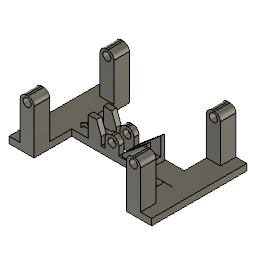
foot (Autodesk Fusion 360 design; units mm, degrees)
part number: 2025-10-24-15-34-12-718
Autodesk Fusion 360 part; units mm, degrees
sketch "Sketch1" plane through (0, 0, 0) normal (0, 0, 1) x (1, 0, 0)
  line L0 (0, 0) -> (180.34, 0)
  line L1 (180.34, 0) -> (180.34, 120.65)
  line L2 (180.34, 120.65) -> (0, 120.65)
  line L3 (0, 120.65) -> (0, 0)
  line L4 (43.18, 0) -> (43.18, 47.625)
  line L5 (43.18, 47.625) -> (137.16, 47.625)
  line L6 (137.16, 47.625) -> (137.16, 0)
  line L7 (43.18, 120.65) -> (43.18, 73.025)
  line L8 (43.18, 73.025) -> (137.16, 73.025)
  line L9 (137.16, 73.025) -> (137.16, 120.65)
  dimension "d1" = 180.34
  dimension "d2" = 120.65
  dimension "d3" = 43.18
  dimension "d4" = 43.18
  dimension "d5" = 43.18
  dimension "d6" = 43.18
  dimension "d8" = 47.625
  dimension "d9" = 47.625
  dimension "d10" = 25.4
  constraint horizontal L0
  constraint vertical L1
  constraint horizontal L2
  constraint vertical L3
  constraint coincident L0.start L3.end
  constraint coincident L0 L4.start
  constraint perpendicular L0 L4
  constraint perpendicular L4 L5
  constraint coincident L0 L6.end
  constraint perpendicular L0 L6
  constraint coincident L2 L7.start
  constraint perpendicular L2 L7
  constraint perpendicular L7 L8
  constraint coincident L2 L9.end
  constraint perpendicular L2 L9
  measures "d1" distance of L0.start L0.end
  measures "d2" distance of L0.start L2.end
  measures "d3" distance of L0.start L4.start
  measures "d4" distance of L0.end L6.end
  measures "d5" distance of L2.end L7.start
  measures "d6" distance of L1.end L9.end
  measures "d8" distance of L8.end L9.end
  measures "d9" distance of L5.end L6.end
  measures "d10" distance of L5.end L8.end
extrude "Extrude1" add sketch "Sketch1" along normal blind 3.175 contours L0 L1 L2 L3 L4 L5 L6 L7 L8 L9
sketch "Sketch2" plane through (0, 0, 3.175) normal (0, 0, 1) x (-1, 0, 0)
  line L0 (-43.18, -120.65) -> (0, -120.65)
  line L1 (0, -120.65) -> (0, 0)
  line L2 (0, 0) -> (-43.18, 0)
  line L3 (-43.18, 0) -> (-43.18, -47.625)
  line L4 (-43.18, -47.625) -> (-137.16, -47.625)
  line L5 (-137.16, -47.625) -> (-137.16, 0)
  line L6 (-137.16, 0) -> (-180.34, 0)
  line L7 (-180.34, 0) -> (-180.34, -120.65)
  line L8 (-180.34, -120.65) -> (-137.16, -120.65)
  line L9 (-137.16, -120.65) -> (-137.16, -73.025)
  line L10 (-137.16, -73.025) -> (-43.18, -73.025)
  line L11 (-43.18, -73.025) -> (-43.18, -120.65)
  line L12 (-73.66, -73.025) -> (-73.66, -47.625)
  line L13 (-91.44, -47.625) -> (-91.44, -73.025)
  dimension "d13" = 30.48
  dimension "d14" = 45.72
  constraint coincident L10 L12.start
  constraint coincident L4 L12.end
  constraint perpendicular L4 L12
  constraint coincident L4 L13.start
  constraint coincident L10 L13.end
  constraint perpendicular L10 L13
  measures "d13" distance of L3.end L12.end
  measures "d14" distance of L4.end L13.start
extrude "Extrude2" add sketch "Sketch2" along normal blind 41.275 contours L4 L10 L12 L13
sketch "Sketch3" plane through (0, 0, 3.175) normal (0, 0, 1) x (-1, 0, 0)
  line L0 (-73.66, -47.625) -> (-73.66, -73.025)
  line L1 (-73.66, -73.025) -> (-43.18, -73.025)
  line L2 (-43.18, -73.025) -> (-43.18, -120.65)
  line L3 (-43.18, -120.65) -> (0, -120.65)
  line L4 (0, -120.65) -> (0, 0)
  line L5 (0, 0) -> (-43.18, 0)
  line L6 (-43.18, 0) -> (-43.18, -47.625)
  line L7 (-43.18, -47.625) -> (-73.66, -47.625)
  line L8 (-31.75, -120.65) -> (-13.97, -120.65)
  line L9 (-13.97, -120.65) -> (-13.97, -100.965)
  line L10 (-13.97, -100.965) -> (-31.75, -100.965)
  line L11 (-31.75, -100.965) -> (-31.75, -120.65)
  line L12 (-31.75, 0) -> (-13.97, 0)
  line L13 (-13.97, 0) -> (-13.97, -19.685)
  line L14 (-13.97, -19.685) -> (-31.75, -19.685)
  line L15 (-31.75, -19.685) -> (-31.75, 0)
  dimension "d18" = 19.685
  dimension "d20" = 19.685
  dimension "d108" = 17.78
  dimension "d109" = 11.43
  dimension "d110" = 17.78
  dimension "d111" = 11.43
  dimension "d113" = 19.685
  constraint horizontal L8
  constraint vertical L9
  constraint horizontal L10
  constraint vertical L11
  constraint horizontal L12
  constraint vertical L13
  constraint horizontal L14
  constraint vertical L15
  constraint coincident L3 L8.start
  measures "d18" distance of L8.start L10.end
  measures "d20" distance of L12.start L14.end
  measures "d108" distance of L9 L11
  measures "d109" distance of L2.end L11
  measures "d110" distance of L13 L15
  measures "d111" distance of L6 L15
  measures "d113" distance of L5 L14
sketch "Sketch4" plane through (0, 0, 3.175) normal (0, 0, 1) x (-1, 0, 0)
  line L0 (-91.44, -73.025) -> (-91.44, -47.625)
  line L1 (-91.44, -47.625) -> (-137.16, -47.625)
  line L2 (-137.16, -47.625) -> (-137.16, 0)
  line L3 (-137.16, 0) -> (-180.34, 0)
  line L4 (-180.34, 0) -> (-180.34, -120.65)
  line L5 (-180.34, -120.65) -> (-137.16, -120.65)
  line L6 (-137.16, -120.65) -> (-137.16, -73.025)
  line L7 (-137.16, -73.025) -> (-91.44, -73.025)
  line L8 (-148.59, -120.65) -> (-166.37, -120.65)
  line L9 (-166.37, -120.65) -> (-166.37, -100.965)
  line L10 (-166.37, -100.965) -> (-148.59, -100.965)
  line L11 (-148.59, 0) -> (-166.37, 0)
  line L12 (-166.37, 0) -> (-166.37, -19.685)
  line L13 (-166.37, -19.685) -> (-148.59, -19.685)
  line L14 (-148.59, -19.685) -> (-148.59, 0)
  line L15 (-148.59, -100.965) -> (-148.59, -120.65)
  dimension "d21" = 17.78
  dimension "d22" = 19.685
  dimension "d95" = 11.43
  dimension "d96" = 17.78
  dimension "d98" = 19.685
  dimension "d99" = 11.43
  constraint horizontal L8
  constraint vertical L9
  constraint horizontal L10
  constraint horizontal L11
  constraint vertical L12
  constraint horizontal L13
  constraint coincident L5 L8.start
  constraint perpendicular L8 L15
  constraint coincident L3 L11.start
  constraint perpendicular L3 L14
  measures "d21" distance of L8.start L8.end
  measures "d22" distance of L8.start L10.end
  measures "d95" distance of L6 L10.end
  measures "d96" distance of L11.start L11.end
  measures "d98" distance of L11.start L13.end
  measures "d99" distance of L2.end L11.start
extrude "Extrude3" add sketch "Sketch3" sketch "Sketch4" along normal blind 41.275 contours L5 L12 L13 L14 L15 | L3 L8 L9 L10 L11 of sketch 2 contours L5 L8 L9 L10 L15 | L3 L11 L12 L13 L14
sketch "Sketch5" plane through (0, 0, 3.175) normal (0, 0, 1) x (-1, 0, 0)
  line L0 (-166.37, -19.685) -> (-166.37, 0)
  line L1 (-166.37, 0) -> (-180.34, 0)
  line L2 (-180.34, 0) -> (-180.34, -120.65)
  line L3 (-180.34, -120.65) -> (-166.37, -120.65)
  line L4 (-166.37, -120.65) -> (-166.37, -100.965)
  line L5 (-166.37, -100.965) -> (-148.59, -100.965)
  line L6 (-137.16, -120.65) -> (-137.16, -73.025)
  line L7 (-137.16, -73.025) -> (-91.44, -73.025)
  line L8 (-91.44, -73.025) -> (-91.44, -47.625)
  line L9 (-91.44, -47.625) -> (-137.16, -47.625)
  line L10 (-137.16, -47.625) -> (-137.16, 0)
  line L11 (-148.59, -19.685) -> (-166.37, -19.685)
  line L12 (-137.16, 0) -> (-158.6586, 0)
  line L13 (-158.6586, 0) -> (-158.6586, -47.6125)
  line L14 (-158.6586, -47.6125) -> (-137.16, -47.6125)
  line L15 (-137.16, -47.6125) -> (-137.16, 0)
  line L16 (-166.37, -100.965) -> (-137.16, -100.965)
  line L17 (-137.16, -100.965) -> (-137.16, -73.025)
  line L18 (-137.16, -73.025) -> (-166.37, -73.025)
  line L19 (-166.37, -73.025) -> (-166.37, -100.965)
  line L20 (-148.59, -100.965) -> (-148.59, -120.65)
  line L21 (-148.59, -120.65) -> (-137.16, -120.65)
  line L22 (-137.16, 0) -> (-148.59, 0)
  line L23 (-148.59, 0) -> (-148.59, -19.685)
  constraint horizontal L12
  constraint vertical L13
  constraint horizontal L14
  constraint vertical L15
  constraint coincident L10.end L12.start
  constraint horizontal L16
  constraint vertical L17
  constraint horizontal L18
  constraint vertical L19
  constraint coincident L6.end L7.start
  constraint coincident L4.end L5.start
sketch "Sketch6" plane through (0, 0, 3.175) normal (0, 0, 1) x (-1, 0, 0)
  line L0 (-13.97, -100.965) -> (-13.97, -120.65)
  line L1 (-13.97, -120.65) -> (0, -120.65)
  line L2 (0, -120.65) -> (0, 0)
  line L3 (0, 0) -> (-13.97, 0)
  line L4 (-13.97, 0) -> (-13.97, -19.685)
  line L5 (-13.97, -19.685) -> (-31.75, -19.685)
  line L6 (-31.75, -19.685) -> (-31.75, 0)
  line L7 (-43.18, -47.625) -> (-73.66, -47.625)
  line L8 (-73.66, -47.625) -> (-73.66, -73.025)
  line L9 (-73.66, -73.025) -> (-43.18, -73.025)
  line L10 (-43.18, -73.025) -> (-43.18, -120.65)
  line L11 (-31.75, -100.965) -> (-13.97, -100.965)
  line L12 (-13.97, -19.685) -> (-31.75, -19.685)
  line L13 (-31.75, -19.685) -> (-31.75, 0)
  line L14 (-31.75, 0) -> (-13.97, 0)
  line L15 (-13.97, 0) -> (-13.97, -19.685)
  line L16 (-13.97, -100.965) -> (-43.18, -100.965)
  line L17 (-43.18, -100.965) -> (-43.18, -73.025)
  line L18 (-43.18, -73.025) -> (-13.97, -73.025)
  line L19 (-13.97, -73.025) -> (-13.97, -100.965)
  line L20 (-31.75, 0) -> (-43.18, 0)
  line L21 (-43.18, 0) -> (-43.18, -47.625)
  line L22 (-43.18, -120.65) -> (-31.75, -120.65)
  line L23 (-31.75, -120.65) -> (-31.75, -100.965)
  constraint horizontal L12
  constraint vertical L13
  constraint horizontal L14
  constraint vertical L15
  constraint coincident L6.end L13.end
  constraint coincident L4.end L5.start
  constraint horizontal L16
  constraint vertical L17
  constraint horizontal L18
  constraint vertical L19
  constraint coincident L9.end L10.start
  constraint coincident L0.start L11.end
extrude "Extrude4" cut sketch "Sketch6" sketch "Sketch5" against normal blind 5.08 contours L10 L11 L16 L17 L18 L19 | L4 L5 L6 L12 L13 L14 L15 of sketch 2 contours L11 L12 L13 L23 | L10 L11 L12 L13 L14 L15 L22 L23 | L5 L6 L16 L17 L18 L19
hole "Hole1" at (82.55, 73.025, 13.335) direction (0, -1, 0) diameter 10.16 depth 30.48 tip angle 118
extrude "Extrude5" add 4 faces at (154.5167, 114.0883, 44.45) (160.4433, 13.1233, 44.45) (25.8233, 6.5617, 44.45) (19.8967, 107.5267, 44.45) along direction (0, 0, 1) blind 14.605
hole "Hole2" at (157.48, 120.65, 51.435) direction (0, -1, 0) diameter 10.16 depth 135.89 tip angle 118
hole "Hole3" at (22.86, 120.65, 51.435) direction (0, -1, 0) diameter 10.16 depth 135.89 tip angle 118
extrude "Extrude6" cut 1 faces at (79.5867, 64.5583, 44.45) along direction (0, 0, -1) blind 22.86
sketch "Sketch7" plane through (0, 0, 21.59) normal (0, 0, 1) x (-1, 0, 0)
  line L0 (-91.44, -47.625) -> (-91.44, -73.025)
  line L1 (-91.44, -73.025) -> (-73.66, -73.025)
  line L2 (-73.66, -73.025) -> (-73.66, -47.625)
  line L3 (-73.66, -47.625) -> (-91.44, -47.625)
  line L4 (-91.44, -53.975) -> (-73.66, -53.975)
  line L5 (-73.66, -53.975) -> (-73.66, -66.675)
  line L6 (-73.66, -66.675) -> (-91.44, -66.675)
  line L7 (-91.44, -66.675) -> (-91.44, -53.975)
  dimension "d48" = 6.35
  dimension "d49" = 6.35
  constraint horizontal L4
  constraint vertical L5
  constraint horizontal L6
  constraint vertical L7
  constraint coincident L2 L5.end
  constraint coincident L0 L4.start
  measures "d48" distance of L3 L4
  measures "d49" distance of L1 L6
extrude "Extrude7" cut sketch "Sketch7" against normal blind 22.86 contours L0 L2 L4 L5 L6 L7
fillet "Fillet1" radius 3.175 1 edges at (73.66, 60.325, 3.175)
fillet "Fillet2" radius 3.175 1 edges at (91.44, 60.325, 3.175)
fillet "Fillet3" radius 7.62 11 edges at (166.37, 9.8425, 59.055) (31.75, 9.8425, 59.055) (31.75, 110.8075, 59.055) (166.37, 110.8075, 59.055) (91.44, 69.85, 21.59) (91.44, 50.8, 21.59) (73.66, 50.8, 21.59) (73.66, 69.85, 21.59) (13.97, 110.8075, 59.055) (13.97, 9.8425, 59.055) (148.59, 9.8425, 59.055)
sketch "Sketch8" plane through (0, 0, 3.175) normal (0, 0, 1) x (-1, 0, 0)
  line L0 (-70.485, -66.675) -> (-73.66, -66.675)
  line L1 (-73.66, -66.675) -> (-73.66, -73.025)
  line L2 (-73.66, -73.025) -> (-13.97, -73.025)
  line L3 (-13.97, -73.025) -> (-13.97, -100.965)
  line L4 (-13.97, -100.965) -> (-13.97, -120.65)
  line L5 (-13.97, -120.65) -> (0, -120.65)
  line L6 (0, -120.65) -> (0, 0)
  line L7 (0, 0) -> (-13.97, 0)
  line L8 (-43.18, -47.625) -> (-73.66, -47.625)
  line L9 (-73.66, -47.625) -> (-73.66, -53.975)
  line L10 (-73.66, -53.975) -> (-70.485, -53.975)
  line L11 (-70.485, -53.975) -> (-70.485, -66.675)
  line L12 (-45.085, -58.3924) -> (-45.085, -62.2024)
  line L13 (-45.085, -62.2024) -> (-36.195, -62.2024)
  line L14 (-36.195, -62.2024) -> (-36.195, -65.7584)
  line L15 (-36.195, -65.7584) -> (-30.732, -60.1732)
  line L16 (-30.732, -60.1732) -> (-36.195, -54.8297)
  line L17 (-36.195, -54.8297) -> (-36.195, -58.3924)
  line L18 (-36.195, -58.3924) -> (-45.085, -58.3924)
  line L19 (-13.97, 0) -> (-13.97, -19.685)
  line L20 (-13.97, -19.685) -> (-31.75, -19.685)
  line L21 (-31.75, -19.685) -> (-31.75, 0)
  line L22 (-31.75, 0) -> (-43.18, 0)
  line L23 (-43.18, 0) -> (-43.18, -47.625)
  dimension "d58" = 4.4726
  dimension "d59" = 3.81
  dimension "d60" = 3.5627
  dimension "d61" = 3.556
  dimension "d62" = 4.4174
  dimension "d75" = 25.4
  constraint parallel L9 L12
  constraint perpendicular L12 L13
  constraint perpendicular L13 L14
  constraint perpendicular L15 L16
  constraint parallel L14 L17
  constraint perpendicular L12 L18
  measures "d58" vertical distance of L0.start L12.end
  measures "d59" distance of L13 L18
  measures "d60" distance of L16.end L17.end
  measures "d61" distance of L13.end L14.end
  measures "d62" vertical distance of L10.end L12.start
  measures "d75" distance of L11 L12.start
extrude "Extrude8" cut sketch "Sketch8" against normal blind 0.508 contours L12 L13 L14 L15 L16 L17 L18
sketch "Sketch9" plane through (0, 0, 3.175) normal (0, 0, 1) x (-1, 0, 0)
  line L0 (-94.615, -53.975) -> (-91.44, -53.975)
  line L1 (-91.44, -53.975) -> (-91.44, -47.625)
  line L2 (-91.44, -47.625) -> (-137.16, -47.625)
  line L3 (-137.16, -47.625) -> (-137.16, -47.6125)
  line L4 (-137.16, -47.6125) -> (-158.6586, -47.6125)
  line L5 (-158.6586, -47.6125) -> (-158.6586, -19.685)
  line L6 (-166.37, -19.685) -> (-166.37, 0)
  line L7 (-166.37, 0) -> (-180.34, 0)
  line L8 (-180.34, 0) -> (-180.34, -120.65)
  line L9 (-180.34, -120.65) -> (-166.37, -120.65)
  line L10 (-166.37, -120.65) -> (-166.37, -100.965)
  line L11 (-166.37, -100.965) -> (-166.37, -73.025)
  line L12 (-166.37, -73.025) -> (-91.44, -73.025)
  line L13 (-91.44, -73.025) -> (-91.44, -66.675)
  line L14 (-91.44, -66.675) -> (-94.615, -66.675)
  line L15 (-94.615, -66.675) -> (-94.615, -53.975)
  line L16 (-107.315, -66.675) -> (-94.615, -66.675)
  line L17 (-94.615, -66.675) -> (-94.615, -53.975)
  line L18 (-94.615, -53.975) -> (-107.315, -53.975)
  line L19 (-107.315, -53.975) -> (-107.315, -66.675)
  line L20 (-158.6586, -19.685) -> (-166.37, -19.685)
  dimension "d65" = 12.7
  dimension "d66" = 12.7
  constraint horizontal L16
  constraint vertical L17
  constraint horizontal L18
  constraint vertical L19
  constraint coincident L0.start L15.end
  measures "d65" distance of L17 L19
  measures "d66" distance of L14.end L0.start
extrude "Extrude9" add sketch "Sketch9" along normal blind 3.7084 contours L15 L16 L17 L18 L19
extrude "Extrude10" cut 1 faces at (103.0817, 58.2083, 6.8834) along direction (0, 0, -1) blind 0.0508
sketch "Sketch10" plane through (0, 66.675, 0) normal (0, 1, 0) x (-1, 0, 0)
  line L0 (-94.615, 6.8326) -> (-107.315, 6.8326)
  line L1 (-107.315, 6.8326) -> (-107.315, 3.175)
  line L2 (-107.315, 3.175) -> (-94.615, 3.175)
  line L3 (-94.615, 3.175) -> (-94.615, 6.8326)
  line L4 (-94.615, 6.8326) -> (-107.315, 17.4892)
  line L5 (-107.315, 17.4892) -> (-107.315, 6.8326)
  dimension "d71" = 90
  dimension "d72" = 40
  constraint coincident L0.start L3.end
  constraint coincident L0.end L1.start
  measures "d71" angle of L0 L5
  measures "d72" angle of L0 L4
extrude "Extrude11" add sketch "Sketch10" against normal blind 12.7 contours L0 L4 L5
sketch "Sketch11" plane through (0, 0, 3.175) normal (0, 0, 1) x (-1, 0, 0)
  line L0 (-45.085, -62.2024) -> (-45.085, -58.3924)
  line L1 (-45.085, -58.3924) -> (-36.195, -58.3924)
  line L2 (-36.195, -58.3924) -> (-36.195, -54.8297)
  line L3 (-36.195, -54.8297) -> (-30.732, -60.1732)
  line L4 (-30.732, -60.1732) -> (-36.195, -65.7584)
  line L5 (-36.195, -65.7584) -> (-36.195, -62.2024)
  line L6 (-36.195, -62.2024) -> (-45.085, -62.2024)
  line L7 (-70.485, -66.675) -> (-73.66, -66.675)
  line L8 (-73.66, -66.675) -> (-73.66, -73.025)
  line L9 (-73.66, -73.025) -> (-13.97, -73.025)
  line L10 (-13.97, -73.025) -> (-13.97, -100.965)
  line L11 (-13.97, -100.965) -> (-13.97, -120.65)
  line L12 (-13.97, -120.65) -> (0, -120.65)
  line L13 (0, -120.65) -> (0, 0)
  line L14 (0, 0) -> (-13.97, 0)
  line L15 (-43.18, -47.625) -> (-73.66, -47.625)
  line L16 (-73.66, -47.625) -> (-73.66, -53.975)
  line L17 (-73.66, -53.975) -> (-70.485, -53.975)
  line L18 (-70.485, -53.975) -> (-70.485, -66.675)
  line L19 (-52.705, -53.975) -> (-70.485, -53.975)
  line L20 (-70.485, -53.975) -> (-70.485, -66.675)
  line L21 (-70.485, -66.675) -> (-52.705, -66.675)
  line L22 (-52.705, -66.675) -> (-52.705, -53.975)
  line L23 (-13.97, 0) -> (-13.97, -19.685)
  line L24 (-13.97, -19.685) -> (-31.75, -19.685)
  line L25 (-31.75, -19.685) -> (-31.75, 0)
  line L26 (-31.75, 0) -> (-43.18, 0)
  line L27 (-43.18, 0) -> (-43.18, -47.625)
  dimension "d76" = 17.78
  dimension "d77" = 12.7
  constraint horizontal L19
  constraint vertical L20
  constraint horizontal L21
  constraint vertical L22
  constraint coincident L7.start L18.end
  measures "d76" distance of L17.end L19.start
  measures "d77" distance of L19.start L21.end
extrude "Extrude12" add sketch "Sketch11" along normal blind 10.16 contours L18 L19 L20 L21 L22
extrude "Extrude13" cut 1 faces at (70.485, 58.2083, 6.5617) along direction (-1, 0, 0) blind 1.27
extrude "Extrude14" cut 1 faces at (69.215, 58.2083, 6.5617) along direction (-1, 0, 0) blind 0.254
sketch "Sketch12" plane through (0, 66.675, 0) normal (0, 1, 0) x (-1, 0, 0)
  line L0 (-68.961, 13.335) -> (-68.961, 3.175)
  line L1 (-68.961, 3.175) -> (-52.705, 3.175)
  line L2 (-52.705, 3.175) -> (-52.705, 13.335)
  line L3 (-52.705, 13.335) -> (-68.961, 13.335)
  line L4 (-68.961, 13.335) -> (-52.705, 57.998)
  line L5 (-52.705, 57.998) -> (-52.705, 13.335)
  dimension "d84" = 90
  dimension "d85" = 70
  constraint coincident L0.start L3.end
  constraint coincident L2.end L3.start
  measures "d84" angle of L3 L5
  measures "d85" angle of L3 L4
extrude "Extrude15" add sketch "Sketch12" against normal blind 12.7 contours L3 L4 L5
sketch "Sketch13" plane through (0, 53.975, 0) normal (0, -1, 0) x (1, 0, 0)
  line L0 (68.961, 3.175) -> (68.961, 13.335)
  line L1 (68.961, 13.335) -> (52.705, 57.998)
  line L2 (52.705, 57.998) -> (52.705, 3.175)
  line L3 (52.705, 3.175) -> (68.961, 3.175)
  line L4 (52.705, 29.125) -> (63.2139, 29.125)
  constraint coincident L2 L4.start
  constraint coincident L1 L4.end
  constraint perpendicular L2 L4
extrude "Extrude16" cut sketch "Sketch13" against normal blind 13.97 contours L1 L2 L4
extrude "Extrude17" add 1 faces at (107.315, 58.2083, 7.9464) along direction (1, 0, 0) blind 17.78
sketch "Sketch14" plane through (0, 53.975, 0) normal (0, -1, 0) x (1, 0, 0)
  line L0 (94.615, 6.8326) -> (94.615, 3.175)
  line L1 (94.615, 3.175) -> (125.095, 3.175)
  line L2 (125.095, 3.175) -> (125.095, 17.4892)
  line L3 (125.095, 17.4892) -> (107.315, 17.4892)
  line L4 (107.315, 17.4892) -> (94.615, 6.8326)
  line L5 (107.315, 17.4892) -> (125.095, 32.4084)
  line L6 (125.095, 32.4084) -> (125.095, 17.4892)
  dimension "d92" = 90
  constraint coincident L3.end L4.start
  constraint parallel L4 L5
  constraint coincident L2.end L3.start
  measures "d92" angle of L3 L6
extrude "Extrude18" add sketch "Sketch14" against normal blind 12.7 contours L3 L5 L6
sketch "Sketch15" plane through (158.6586, 0, 0) normal (-1, 0, 0) x (0, -1, 0)
  line L0 (-47.6125, 0) -> (0, 0)
  line L1 (0, 0) -> (0, 3.175)
  line L2 (0, 3.175) -> (-19.685, 3.175)
  line L3 (-19.685, 3.175) -> (-47.6125, 3.175)
  line L4 (-47.6125, 3.175) -> (-47.6125, 0)
  line L5 (-19.685, 3.175) -> (0, 3.175)
  line L6 (0, 3.175) -> (0, 0)
  line L7 (0, 0) -> (-19.685, 0)
  line L8 (-19.685, 0) -> (-19.685, 3.175)
  constraint horizontal L5
  constraint vertical L6
  constraint horizontal L7
  constraint vertical L8
  constraint coincident L0.end L1.start
  constraint coincident L2.end L3.start
extrude "Extrude19" add sketch "Sketch15" along normal blind 21.59 contours L0 L1 L2 L5 L6 L7 L8
extrude "Extrude20" cut 1 faces at (137.0686, 13.1233, 2.1167) along direction (1, 0, 0) blind 11.43
extrude "Extrude21" cut 1 faces at (137.16, 114.0883, 2.1167) along direction (1, 0, 0) blind 11.43
extrude "Extrude22" cut 1 faces at (148.4986, 13.1233, 2.1167) along direction (1, 0, 0) blind 0.094
extrude "Extrude23" add 1 faces at (25.8233, 19.685, 2.1167) along direction (0, -1, 0) blind 19.685
fillet "Fillet4" radius 7.62 1 edges at (148.59, 110.8075, 59.055)
sketch "Sketch16" plane through (0, 0, 3.175) normal (0, 0, 1) x (-1, 0, 0)
  line L0 (-68.961, -53.975) -> (-52.705, -53.975)
  line L1 (-52.705, -53.975) -> (-52.705, -66.675)
  line L2 (-52.705, -66.675) -> (-68.961, -66.675)
  line L3 (-68.961, -66.675) -> (-68.961, -53.975)
  line L4 (-70.485, -53.975) -> (-70.485, -66.675)
  line L5 (-70.485, -66.675) -> (-73.66, -66.675)
  line L6 (-73.66, -66.675) -> (-73.66, -73.025)
  line L7 (-73.66, -73.025) -> (-13.97, -73.025)
  line L8 (-13.97, -73.025) -> (-13.97, -100.965)
  line L9 (-13.97, -100.965) -> (-13.97, -120.65)
  line L10 (-13.97, -120.65) -> (0, -120.65)
  line L11 (0, -120.65) -> (0, 0)
  line L12 (0, 0) -> (-13.97, 0)
  line L13 (-13.97, 0) -> (-13.97, -19.685)
  line L14 (-13.97, -19.685) -> (-31.75, -19.685)
  line L15 (-31.75, -19.685) -> (-31.75, 0)
  line L16 (-31.75, 0) -> (-43.18, 0)
  line L17 (-43.18, 0) -> (-43.18, -47.625)
  line L18 (-43.18, -47.625) -> (-73.66, -47.625)
  line L19 (-73.66, -47.625) -> (-73.66, -53.975)
  line L20 (-73.66, -53.975) -> (-70.485, -53.975)
  line L21 (-45.085, -62.2024) -> (-45.085, -58.3924)
  line L22 (-45.085, -58.3924) -> (-36.195, -58.3924)
  line L23 (-36.195, -58.3924) -> (-36.195, -54.8297)
  line L24 (-36.195, -54.8297) -> (-30.732, -60.1732)
  line L25 (-30.732, -60.1732) -> (-36.195, -65.7584)
  line L26 (-36.195, -65.7584) -> (-36.195, -62.2024)
  line L27 (-36.195, -62.2024) -> (-45.085, -62.2024)
  line L28 (-43.18, -47.625) -> (-31.75, -47.625)
  line L29 (-31.75, -47.625) -> (-31.75, 0)
  line L30 (-31.75, 0) -> (-43.18, 0)
  line L31 (-43.18, 0) -> (-43.18, -47.625)
  constraint horizontal L28
  constraint vertical L29
  constraint horizontal L30
  constraint vertical L31
  constraint coincident L15.end L16.start
  constraint coincident L17.end L18.start
extrude "Extrude24" cut sketch "Sketch16" against normal blind 10.16 contours L15 L16 L17 L28 L29 L30 L31
extrude "Extrude25" cut 1 faces at (35.56, 114.0883, 3.175) along direction (0, 0, -1) blind 7.62
sketch "Sketch17" plane through (125.095, 0, 0) normal (1, 0, 0) x (0, 1, 0)
  line L0 (53.975, 32.4084) -> (53.975, 3.175)
  line L1 (53.975, 3.175) -> (66.675, 3.175)
  line L2 (66.675, 3.175) -> (66.675, 32.4084)
  line L3 (66.675, 32.4084) -> (53.975, 32.4084)
  line L4 (57.15, 32.4084) -> (63.5, 32.4084)
  line L5 (63.5, 32.4084) -> (63.5, 13.97)
  line L6 (63.5, 13.97) -> (57.15, 13.97)
  line L7 (57.15, 13.97) -> (57.15, 32.4084)
  dimension "d122" = 6.35
  dimension "d123" = 12.7
  dimension "d124" = 3.175
  dimension "d125" = 3.175
  constraint horizontal L4
  constraint vertical L5
  constraint horizontal L6
  constraint vertical L7
  constraint coincident L3 L4.start
  measures "d122" distance of L4.start L4.end
  measures "d123" distance of L0.start L2.end
  measures "d124" distance of L0.start L4.start
  measures "d125" distance of L2.end L4.end
extrude "Extrude26" cut sketch "Sketch17" against normal blind 78.74 contours L3 L4 L5 L6 L7
extrude "Extrude27" add 1 faces at (58.1237, 53.975, 15.2117) along direction (0, -1, 0) blind 5.08
extrude "Extrude28" add 1 faces at (58.1237, 66.675, 15.2117) along direction (0, 1, 0) blind 5.08
sketch "Sketch18" plane through (52.705, 0, 0) normal (-1, 0, 0) x (0, -1, 0)
  line L0 (-63.5, 13.97) -> (-63.5, 29.125)
  line L1 (-63.5, 29.125) -> (-71.755, 29.125)
  line L2 (-71.755, 29.125) -> (-71.755, 3.175)
  line L3 (-71.755, 3.175) -> (-48.895, 3.175)
  line L4 (-48.895, 3.175) -> (-48.895, 29.125)
  line L5 (-48.895, 29.125) -> (-57.15, 29.125)
  line L6 (-57.15, 29.125) -> (-57.15, 13.97)
  line L7 (-57.15, 13.97) -> (-63.5, 13.97)
  line L8 (-66.675, 29.125) -> (-66.675, 13.97)
  line L9 (-66.675, 13.97) -> (-66.675, 6.35)
  line L10 (-66.675, 6.35) -> (-53.975, 6.35)
  line L11 (-53.975, 6.35) -> (-53.975, 29.125)
  dimension "d132" = 6.35
  dimension "d133" = 90
  dimension "d134" = 90
  dimension "d136" = 12.7
  dimension "d137" = 22.86
  dimension "d138" = 5.08
  constraint perpendicular L1 L8
  constraint perpendicular L3 L9
  constraint perpendicular L9 L10
  measures "d132" distance of L0.end L5.end
  measures "d133" angle of L9 L10
  measures "d134" angle of L10 L11
  measures "d136" distance of L9 L11
  measures "d137" distance of L1.end L4.end
  measures "d138" distance of L1.end L8.start
extrude "Extrude29" cut sketch "Sketch18" against normal blind 17.78 contours L0 L1 L5 L6 L7 L8 L9 L10 L11
extrude "Extrude30" add 1 faces at (114.935, 53.975, 14.1387) along direction (0, -1, 0) blind 5.08
extrude "Extrude31" add 1 faces at (114.935, 66.675, 14.1387) along direction (0, 1, 0) blind 5.08
extrude "Extrude33" add 1 faces at (58.1237, 71.755, 15.2117) along direction (0, 1, 0) blind 1.27
extrude "Extrude34" add 1 faces at (58.1237, 48.895, 15.2117) along direction (0, -1, 0) blind 1.27
sketch "Sketch20" plane through (125.095, 0, 0) normal (1, 0, 0) x (0, 1, 0)
  line L0 (57.15, 13.97) -> (57.15, 32.4084)
  line L1 (57.15, 32.4084) -> (48.895, 32.4084)
  line L2 (48.895, 32.4084) -> (48.895, 3.175)
  line L3 (48.895, 3.175) -> (71.755, 3.175)
  line L4 (71.755, 3.175) -> (71.755, 32.4084)
  line L5 (71.755, 32.4084) -> (63.5, 32.4084)
  line L6 (63.5, 32.4084) -> (63.5, 13.97)
  line L7 (63.5, 13.97) -> (57.15, 13.97)
  line L8 (53.975, 32.4084) -> (53.975, 9.6246)
  line L9 (53.975, 9.6246) -> (66.675, 9.6246)
  line L10 (66.675, 9.6246) -> (66.675, 32.4084)
  dimension "d151" = 22.7838
  dimension "d152" = 12.7
  dimension "d153" = 5.08
  constraint perpendicular L3 L8
  constraint perpendicular L8 L9
  constraint coincident L5 L10.end
  constraint perpendicular L5 L10
  measures "d151" distance of L8.start L8.end
  measures "d152" distance of L8.end L9.end
  measures "d153" distance of L1.end L8.start
extrude "Extrude35" cut sketch "Sketch20" against normal blind 30.48 contours L0 L1 L5 L6 L7 L8 L9 L10
extrude "Extrude36" add 3 faces at (21.1667, 15.875, 0) (73.66, 58.2083, 0.0002) (91.44, 58.2083, 0.0004) along direction (0, 0, -1) blind 5.08
sketch "Sketch21" plane through (0, 100.965, 0) normal (0, -1, 0) x (1, 0, 0)
  arc A0 (156.21, 59.055) -> (148.59, 51.435) centre (156.21, 51.435) ccw
  line L0 (148.59, 51.435) -> (148.59, -5.08)
  line L1 (148.59, -5.08) -> (166.37, -5.08)
  line L2 (166.37, -5.08) -> (166.37, 3.175)
  line L3 (166.37, 3.175) -> (166.37, 51.435)
  arc A1 (166.37, 51.435) -> (158.75, 59.055) centre (158.75, 51.435) ccw
  line L4 (158.75, 59.055) -> (156.21, 59.055)
  circle A2 centre (157.48, 51.435) radius 5.08
  line L5 (166.37, 3.175) -> (148.59, 3.175)
  line L6 (148.59, 3.175) -> (148.59, -5.08)
  line L7 (148.59, -5.08) -> (166.37, -5.08)
  line L8 (166.37, -5.08) -> (166.37, 3.175)
  line L9 (13.97, -5.08) -> (31.75, -5.08)
  line L10 (31.75, -5.08) -> (31.75, 2.54)
  line L11 (31.75, 2.54) -> (13.97, 2.54)
  line L12 (13.97, 2.54) -> (13.97, -5.08)
  constraint horizontal L5
  constraint vertical L6
  constraint horizontal L7
  constraint vertical L8
  constraint coincident L0.end L1.start
  constraint coincident L2.end L3.start
  constraint horizontal L9
  constraint vertical L10
  constraint horizontal L11
  constraint vertical L12
extrude "Extrude37" add sketch "Sketch21" along normal blind 27.94 contours L0 L1 L2 L5 L6 L7 L8 | L9 L10 L11 L12
extrude "Extrude38" add 1 faces at (25.8233, 91.6517, 2.54) along direction (0, 0, 1) blind 0.635
sketch "Sketch22" plane through (0, 19.685, 0) normal (0, 1, 0) x (-1, 0, 0)
  line L0 (-148.5926, 3.175) -> (-148.59, 3.175)
  line L1 (-148.59, 3.175) -> (-148.59, 51.435)
  arc A0 (-148.59, 51.435) -> (-156.21, 59.055) centre (-156.21, 51.435) ccw
  line L2 (-156.21, 59.055) -> (-158.75, 59.055)
  arc A1 (-158.75, 59.055) -> (-166.37, 51.435) centre (-158.75, 51.435) ccw
  line L3 (-166.37, 51.435) -> (-166.37, 3.175)
  line L4 (-166.37, 3.175) -> (-158.6586, 3.175)
  line L5 (-158.6586, 3.175) -> (-158.6586, -5.08)
  line L6 (-158.6586, -5.08) -> (-148.5926, -5.08)
  line L7 (-148.5926, -5.08) -> (-148.5926, 3.175)
  circle A2 centre (-157.48, 51.435) radius 5.08
  line L8 (-158.6586, 3.175) -> (-148.5926, 3.175)
  line L9 (-148.5926, 3.175) -> (-148.5926, -5.08)
  line L10 (-148.5926, -5.08) -> (-158.6586, -5.08)
  line L11 (-158.6586, -5.08) -> (-158.6586, 3.175)
  constraint horizontal L8
  constraint vertical L9
  constraint horizontal L10
  constraint vertical L11
  constraint coincident L6.end L7.start
  constraint coincident L4.end L5.start
extrude "Extrude39" add sketch "Sketch22" along normal blind 27.9273 contours L5 L6 L7 L8 L9 L10 L11
equation "d2 = 4 3/4\""
equation "d8 = 1 7/8\""
equation "d11 = ( 1 / 8 ) * 1 in"
equation "d15 = 1 5/8\""
equation "d18 = 0.4 in + ( 3 / 8 ) * 1 in"
equation "d20 = 0.4 in + 0.375 in"
equation "d22 = 0.4 in + 0.375 in"
equation "d25 = 1 in + ( 5 / 8 ) * 1 in"
equation "d33 = ( ( 1 / 8 ) * 1 in ) + 0.4 in"
equation "d98 = 0.4 in + 0.375 in"
